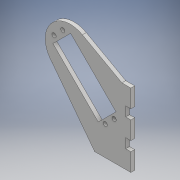
# Autodesk Inventor part: planos robot
Saved by Autodesk Inventor 2018 (Build 220112000, 112)
## iProperties
Created: 2020-03-10
Part Number: planos robot
Material: Genérico
Document SubType Name: Modeling
Designer: sala.ceri
Density: 1 g/cm^3
Appearance: Valor por defecto
Author: sala.ceri
Autodesk Inventor part; units mm, degrees
ref_plane "YZ Plane" through (0, 0, 0) normal (1, 0, 0) x (0, 1, 0)
ref_plane "XZ Plane" through (0, 0, 0) normal (0, 1, 0) x (-1, 0, 0)
ref_plane "XY Plane" through (0, 0, 0) normal (0, 0, 1) x (1, 0, 0)
sketch "Boceto1" plane through (0, 0, 0) normal (0, 1, 0) x (-1, 0, 0)
  line L0 (13.5057, -0.2828) -> (-21.8496, -35.6382)
  line L1 (13.5057, -0.2828) -> (-0.2828, 13.5057)
  line L2 (-0.2828, 13.5057) -> (-35.6382, -21.8496)
  line L3 (-35.6382, -21.8496) -> (-21.8496, -35.6382)
  circle A0 centre (12.6395, 5.7452) radius 1.65
  circle A1 centre (5.7452, 12.6395) radius 1.65
  circle A2 centre (-27.312, -34.2063) radius 1.65
  circle A3 centre (-34.2063, -27.312) radius 1.65
  arc A4 (14.2895, -13.2687) -> (-9.4509, 17.0567) centre (0, 0) ccw
  line L4 (-40.2344, 0) -> (-9.4509, 17.0567)
  line L5 (-40.2344, 0) -> (-43.2344, 0)
  line L6 (-19.0256, -57) -> (14.2895, -13.2687)
  line L7 (-43.2344, -57) -> (-19.0256, -57)
  line L8 (-43.2344, 0) -> (-47.2344, 0)
  line L9 (-47.2344, 0) -> (-47.2344, -14)
  line L10 (-47.2344, -14) -> (-43.2344, -14)
  line L11 (-43.2344, -57) -> (-47.2344, -57)
  line L12 (-47.2344, -57) -> (-47.2344, -43)
  line L13 (-47.2344, -43) -> (-43.2344, -43)
  line L14 (-47.2344, -21.5) -> (-43.2344, -21.5)
  line L15 (-47.2344, -21.5) -> (-47.2344, -35.5)
  line L16 (-47.2344, -35.5) -> (-43.2344, -35.5)
  line L17 (-43.2344, -14) -> (-43.2344, -21.5)
  line L18 (-43.2344, -35.5) -> (-43.2344, -43)
  dimension "d17" = 3
  dimension "d21" = 14
  dimension "d22" = 14
  dimension "d25" = 14
  dimension "d109" = 7.5
  dimension "d110" = 7.5
  dimension "d111" = 4
  dimension "d112" = 57
  constraints: 38 end point, 12 perpendicular, 5 centre point, 4 vertical, 2 horizontal, 2 point on circle, 1 tangent
  measures "d17" distance of L4.start L5.end
  measures "d21" distance of L8.end L9.end
  measures "d22" distance of L11.end L12.end
  measures "d25" distance of L14.start L15.end
  measures "d109" distance of L10.end L14.end
  measures "d110" distance of L16.end L13.end
  measures "d111" distance of L12.end L13.end
  measures "d112" distance between parallel lines of L11 L8
extrude "Extrusión1" add sketch "Boceto1" along normal blind 3
